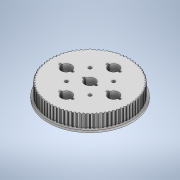
# Autodesk Inventor part: os_5_zebatka
Saved by Autodesk Inventor 2020.3 (Build 243373000, 373)
## iProperties
Created: 2021-03-12
Part Number: os_5_zebatka
Material: Generic
Document SubType Name: Modeling
Designer: patry
Density: 1 g/cm^3
Appearance: Default
Author: patry
Autodesk Inventor part; units mm, degrees
ref_plane "YZ Plane" through (0, 0, 0) normal (1, 0, 0) x (0, 1, 0)
ref_plane "XZ Plane" through (0, 0, 0) normal (0, 1, 0) x (-1, 0, 0)
ref_plane "XY Plane" through (0, 0, 0) normal (0, 0, 1) x (1, 0, 0)
sketch "Sketch1" plane through (0, 0, 0) normal (0, 1, 0) x (-1, 0, 0)
  circle A0 centre (0, 0) radius 40
  dimension "d0" = 80
  constraints: 1 centre point, 1 coincident
  measures "d0" diameter of A0
extrude "Extrusion1" add sketch "Sketch1" along normal blind 2
sketch "Sketch2" plane through (0, 2, 0) normal (0, 1, 0) x (1, 0, 0)
  circle A0 centre (0, 0) radius 38
  line L0 (0.3625, 37.9999) -> (-0.3625, 37.9999)
  arc A1 (-1.5, 36.8624) -> (-0.5625, 37.7999) centre (-1.5, 37.7999) ccw
  arc A2 (0.5625, 37.7999) -> (1.5, 36.8624) centre (1.5, 37.7999) ccw
  arc A3 (-0.3625, 37.9999) -> (-0.5625, 37.7999) centre (-0.3625, 37.7999) ccw
  arc A4 (0.5625, 37.7999) -> (0.3625, 37.9999) centre (0.3625, 37.7999) ccw
  arc A5 (-4.3876, 36.6311) -> (-3.5265, 37.6393) centre (-4.4611, 37.5657) ccw
  arc A6 (-3.3428, 37.8543) -> (-3.5265, 37.6393) centre (-3.3271, 37.655) ccw
  line L1 (-2.6201, 37.9112) -> (-3.3428, 37.8543)
  arc A7 (-2.405, 37.7275) -> (-2.6201, 37.9112) centre (-2.6044, 37.7118) ccw
  arc A8 (-2.405, 37.7275) -> (-1.3968, 36.8665) centre (-1.4704, 37.8011) ccw
  arc A9 (-7.2481, 36.1739) -> (-6.4688, 37.2465) centre (-7.3947, 37.0999) ccw
  arc A10 (-6.3025, 37.4754) -> (-6.4688, 37.2465) centre (-6.2712, 37.2778) ccw
  line L2 (-5.5865, 37.5888) -> (-6.3025, 37.4754)
  arc A11 (-5.3576, 37.4225) -> (-5.5865, 37.5888) centre (-5.5552, 37.3912) ccw
  arc A12 (-5.3576, 37.4225) -> (-4.285, 36.6432) centre (-4.4317, 37.5692) ccw
  arc A13 (-10.0639, 35.4937) -> (-9.3712, 36.6242) centre (-10.2828, 36.4053) ccw
  arc A14 (-9.2234, 36.8654) -> (-9.3712, 36.6242) centre (-9.1767, 36.6709) ccw
  line L3 (-8.5184, 37.0346) -> (-9.2234, 36.8654)
  arc A15 (-8.2773, 36.8868) -> (-8.5184, 37.0346) centre (-8.4717, 36.8401) ccw
  arc A16 (-8.2773, 36.8868) -> (-7.1468, 36.1941) centre (-7.3657, 37.1057) ccw
  arc A17 (-12.8177, 34.5947) -> (-12.2158, 35.776) centre (-13.1074, 35.4863) ccw
  arc A18 (-12.0874, 36.0281) -> (-12.2158, 35.776) centre (-12.0256, 35.8378) ccw
  line L4 (-11.3979, 36.2521) -> (-12.0874, 36.0281)
  arc A19 (-11.1458, 36.1237) -> (-11.3979, 36.2521) centre (-11.3361, 36.0619) ccw
  arc A20 (-11.1458, 36.1237) -> (-9.9645, 35.5218) centre (-10.2542, 36.4134) ccw
  arc A21 (-15.4925, 33.4824) -> (-14.9851, 34.7073) centre (-15.8512, 34.3485) ccw
  arc A22 (-14.8768, 34.9686) -> (-14.9851, 34.7073) centre (-14.8003, 34.7839) ccw
  line L5 (-14.207, 35.2461) -> (-14.8768, 34.9686)
  arc A23 (-13.9457, 35.1378) -> (-14.207, 35.2461) centre (-14.1305, 35.0613) ccw
  arc A24 (-13.9457, 35.1378) -> (-12.7208, 34.6305) centre (-13.0796, 35.4966) ccw
  arc A25 (-18.0717, 32.1637) -> (-17.662, 33.4246) centre (-18.4973, 32.999) ccw
  arc A26 (-17.5746, 33.6936) -> (-17.662, 33.4246) centre (-17.4838, 33.5154) ccw
  line L6 (-16.9286, 34.0227) -> (-17.5746, 33.6936)
  arc A27 (-16.6596, 33.9353) -> (-16.9286, 34.0227) centre (-16.8378, 33.8445) ccw
  arc A28 (-16.6596, 33.9353) -> (-15.3987, 33.5256) centre (-15.8243, 34.361) ccw
  arc A29 (-20.5395, 30.6466) -> (-20.23, 31.9358) centre (-21.0294, 31.446) ccw
  arc A30 (-20.164, 32.2109) -> (-20.23, 31.9358) centre (-20.0595, 32.0403) ccw
  line L7 (-19.5458, 32.5897) -> (-20.164, 32.2109)
  arc A31 (-19.2708, 32.5236) -> (-19.5458, 32.5897) centre (-19.4413, 32.4191) ccw
  arc A32 (-19.2708, 32.5236) -> (-17.9816, 32.2141) centre (-18.4714, 33.0135) ccw
  arc A33 (-22.8807, 28.9406) -> (-22.6733, 30.2501) centre (-23.4318, 29.6991) ccw
  arc A34 (-22.6291, 30.5295) -> (-22.6733, 30.2501) centre (-22.5115, 30.3677) ccw
  line L8 (-22.0425, 30.9557) -> (-22.6291, 30.5295)
  arc A35 (-21.7632, 30.9114) -> (-22.0425, 30.9557) centre (-21.925, 30.7939) ccw
  arc A36 (-21.7632, 30.9114) -> (-20.4537, 30.704) centre (-21.0047, 31.4625) ccw
  arc A37 (-25.0808, 27.0562) -> (-24.9768, 28.378) centre (-25.6897, 27.7691) ccw
  arc A38 (-24.9546, 28.6599) -> (-24.9768, 28.378) centre (-24.8247, 28.5079) ccw
  line L9 (-24.4033, 29.1308) -> (-24.9546, 28.6599)
  arc A39 (-24.1214, 29.1086) -> (-24.4033, 29.1308) centre (-24.2734, 28.9787) ccw
  arc A40 (-24.1214, 29.1086) -> (-22.7996, 29.0046) centre (-23.4085, 29.7175) ccw
  arc A41 (-27.1263, 25.005) -> (-27.1263, 26.3308) centre (-27.7892, 25.6679) ccw
  arc A42 (-27.1263, 26.6137) -> (-27.1263, 26.3308) centre (-26.9849, 26.4723) ccw
  line L10 (-26.6137, 27.1263) -> (-27.1263, 26.6137)
  arc A43 (-26.3308, 27.1263) -> (-26.6137, 27.1263) centre (-26.4723, 26.9849) ccw
  arc A44 (-26.3308, 27.1263) -> (-25.005, 27.1263) centre (-25.6679, 27.7892) ccw
  arc A45 (-29.0046, 22.7996) -> (-29.1086, 24.1214) centre (-29.7175, 23.4085) ccw
  arc A46 (-29.1308, 24.4033) -> (-29.1086, 24.1214) centre (-28.9787, 24.2734) ccw
  line L11 (-28.6599, 24.9546) -> (-29.1308, 24.4033)
  arc A47 (-28.378, 24.9768) -> (-28.6599, 24.9546) centre (-28.5079, 24.8247) ccw
  arc A48 (-28.378, 24.9768) -> (-27.0562, 25.0808) centre (-27.7691, 25.6897) ccw
  arc A49 (-30.704, 20.4537) -> (-30.9114, 21.7632) centre (-31.4625, 21.0047) ccw
  arc A50 (-30.9557, 22.0425) -> (-30.9114, 21.7632) centre (-30.7939, 21.925) ccw
  line L12 (-30.5295, 22.6291) -> (-30.9557, 22.0425)
  arc A51 (-30.2501, 22.6733) -> (-30.5295, 22.6291) centre (-30.3677, 22.5115) ccw
  arc A52 (-30.2501, 22.6733) -> (-28.9406, 22.8807) centre (-29.6991, 23.4318) ccw
  arc A53 (-32.2141, 17.9816) -> (-32.5236, 19.2708) centre (-33.0135, 18.4714) ccw
  arc A54 (-32.5897, 19.5458) -> (-32.5236, 19.2708) centre (-32.4191, 19.4413) ccw
  line L13 (-32.2109, 20.164) -> (-32.5897, 19.5458)
  arc A55 (-31.9358, 20.23) -> (-32.2109, 20.164) centre (-32.0403, 20.0595) ccw
  arc A56 (-31.9358, 20.23) -> (-30.6466, 20.5395) centre (-31.446, 21.0294) ccw
  arc A57 (-33.5256, 15.3987) -> (-33.9353, 16.6596) centre (-34.361, 15.8243) ccw
  arc A58 (-34.0227, 16.9286) -> (-33.9353, 16.6596) centre (-33.8445, 16.8378) ccw
  line L14 (-33.6936, 17.5746) -> (-34.0227, 16.9286)
  arc A59 (-33.4246, 17.662) -> (-33.6936, 17.5746) centre (-33.5154, 17.4838) ccw
  arc A60 (-33.4246, 17.662) -> (-32.1637, 18.0717) centre (-32.999, 18.4973) ccw
  arc A61 (-34.6305, 12.7208) -> (-35.1378, 13.9457) centre (-35.4966, 13.0796) ccw
  arc A62 (-35.2461, 14.207) -> (-35.1378, 13.9457) centre (-35.0613, 14.1305) ccw
  line L15 (-34.9686, 14.8768) -> (-35.2461, 14.207)
  arc A63 (-34.7073, 14.9851) -> (-34.9686, 14.8768) centre (-34.7839, 14.8003) ccw
  arc A64 (-34.7073, 14.9851) -> (-33.4824, 15.4925) centre (-34.3485, 15.8512) ccw
  arc A65 (-35.5218, 9.9645) -> (-36.1237, 11.1458) centre (-36.4134, 10.2542) ccw
  arc A66 (-36.2521, 11.3979) -> (-36.1237, 11.1458) centre (-36.0619, 11.3361) ccw
  line L16 (-36.0281, 12.0874) -> (-36.2521, 11.3979)
  arc A67 (-35.776, 12.2158) -> (-36.0281, 12.0874) centre (-35.8378, 12.0256) ccw
  arc A68 (-35.776, 12.2158) -> (-34.5947, 12.8177) centre (-35.4863, 13.1074) ccw
  arc A69 (-36.1941, 7.1468) -> (-36.8868, 8.2773) centre (-37.1057, 7.3657) ccw
  arc A70 (-37.0346, 8.5184) -> (-36.8868, 8.2773) centre (-36.8401, 8.4717) ccw
  line L17 (-36.8654, 9.2234) -> (-37.0346, 8.5184)
  arc A71 (-36.6242, 9.3712) -> (-36.8654, 9.2234) centre (-36.6709, 9.1767) ccw
  arc A72 (-36.6242, 9.3712) -> (-35.4937, 10.0639) centre (-36.4053, 10.2828) ccw
  arc A73 (-36.6432, 4.285) -> (-37.4225, 5.3576) centre (-37.5692, 4.4317) ccw
  arc A74 (-37.5888, 5.5865) -> (-37.4225, 5.3576) centre (-37.3912, 5.5552) ccw
  line L18 (-37.4754, 6.3025) -> (-37.5888, 5.5865)
  arc A75 (-37.2465, 6.4688) -> (-37.4754, 6.3025) centre (-37.2778, 6.2712) ccw
  arc A76 (-37.2465, 6.4688) -> (-36.1739, 7.2481) centre (-37.0999, 7.3947) ccw
  arc A77 (-36.8665, 1.3968) -> (-37.7275, 2.405) centre (-37.8011, 1.4704) ccw
  arc A78 (-37.9112, 2.6201) -> (-37.7275, 2.405) centre (-37.7118, 2.6044) ccw
  line L19 (-37.8543, 3.3428) -> (-37.9112, 2.6201)
  arc A79 (-37.6393, 3.5265) -> (-37.8543, 3.3428) centre (-37.655, 3.3271) ccw
  arc A80 (-37.6393, 3.5265) -> (-36.6311, 4.3876) centre (-37.5657, 4.4611) ccw
  arc A81 (-36.8624, -1.5) -> (-37.7999, -0.5625) centre (-37.7999, -1.5) ccw
  arc A82 (-37.9999, -0.3625) -> (-37.7999, -0.5625) centre (-37.7999, -0.3625) ccw
  line L20 (-37.9999, 0.3625) -> (-37.9999, -0.3625)
  arc A83 (-37.7999, 0.5625) -> (-37.9999, 0.3625) centre (-37.7999, 0.3625) ccw
  arc A84 (-37.7999, 0.5625) -> (-36.8624, 1.5) centre (-37.7999, 1.5) ccw
  arc A85 (-36.6311, -4.3876) -> (-37.6393, -3.5265) centre (-37.5657, -4.4611) ccw
  arc A86 (-37.8543, -3.3428) -> (-37.6393, -3.5265) centre (-37.655, -3.3271) ccw
  line L21 (-37.9112, -2.6201) -> (-37.8543, -3.3428)
  arc A87 (-37.7275, -2.405) -> (-37.9112, -2.6201) centre (-37.7118, -2.6044) ccw
  arc A88 (-37.7275, -2.405) -> (-36.8665, -1.3968) centre (-37.8011, -1.4704) ccw
  arc A89 (-36.1739, -7.2481) -> (-37.2465, -6.4688) centre (-37.0999, -7.3947) ccw
  arc A90 (-37.4754, -6.3025) -> (-37.2465, -6.4688) centre (-37.2778, -6.2712) ccw
  line L22 (-37.5888, -5.5865) -> (-37.4754, -6.3025)
  arc A91 (-37.4225, -5.3576) -> (-37.5888, -5.5865) centre (-37.3912, -5.5552) ccw
  arc A92 (-37.4225, -5.3576) -> (-36.6432, -4.285) centre (-37.5692, -4.4317) ccw
  arc A93 (-35.4937, -10.0639) -> (-36.6242, -9.3712) centre (-36.4053, -10.2828) ccw
  arc A94 (-36.8654, -9.2234) -> (-36.6242, -9.3712) centre (-36.6709, -9.1767) ccw
  line L23 (-37.0346, -8.5184) -> (-36.8654, -9.2234)
  arc A95 (-36.8868, -8.2773) -> (-37.0346, -8.5184) centre (-36.8401, -8.4717) ccw
  arc A96 (-36.8868, -8.2773) -> (-36.1941, -7.1468) centre (-37.1057, -7.3657) ccw
  arc A97 (-34.5947, -12.8177) -> (-35.776, -12.2158) centre (-35.4863, -13.1074) ccw
  arc A98 (-36.0281, -12.0874) -> (-35.776, -12.2158) centre (-35.8378, -12.0256) ccw
  line L24 (-36.2521, -11.3979) -> (-36.0281, -12.0874)
  arc A99 (-36.1237, -11.1458) -> (-36.2521, -11.3979) centre (-36.0619, -11.3361) ccw
  arc A100 (-36.1237, -11.1458) -> (-35.5218, -9.9645) centre (-36.4134, -10.2542) ccw
  arc A101 (-33.4824, -15.4925) -> (-34.7073, -14.9851) centre (-34.3485, -15.8512) ccw
  arc A102 (-34.9686, -14.8768) -> (-34.7073, -14.9851) centre (-34.7839, -14.8003) ccw
  line L25 (-35.2461, -14.207) -> (-34.9686, -14.8768)
  arc A103 (-35.1378, -13.9457) -> (-35.2461, -14.207) centre (-35.0613, -14.1305) ccw
  arc A104 (-35.1378, -13.9457) -> (-34.6305, -12.7208) centre (-35.4966, -13.0796) ccw
  arc A105 (-32.1637, -18.0717) -> (-33.4246, -17.662) centre (-32.999, -18.4973) ccw
  arc A106 (-33.6936, -17.5746) -> (-33.4246, -17.662) centre (-33.5154, -17.4838) ccw
  line L26 (-34.0227, -16.9286) -> (-33.6936, -17.5746)
  arc A107 (-33.9353, -16.6596) -> (-34.0227, -16.9286) centre (-33.8445, -16.8378) ccw
  arc A108 (-33.9353, -16.6596) -> (-33.5256, -15.3987) centre (-34.361, -15.8243) ccw
  arc A109 (-30.6466, -20.5395) -> (-31.9358, -20.23) centre (-31.446, -21.0294) ccw
  arc A110 (-32.2109, -20.164) -> (-31.9358, -20.23) centre (-32.0403, -20.0595) ccw
  line L27 (-32.5897, -19.5458) -> (-32.2109, -20.164)
  arc A111 (-32.5236, -19.2708) -> (-32.5897, -19.5458) centre (-32.4191, -19.4413) ccw
  arc A112 (-32.5236, -19.2708) -> (-32.2141, -17.9816) centre (-33.0135, -18.4714) ccw
  arc A113 (-28.9406, -22.8807) -> (-30.2501, -22.6733) centre (-29.6991, -23.4318) ccw
  arc A114 (-30.5295, -22.6291) -> (-30.2501, -22.6733) centre (-30.3677, -22.5115) ccw
  line L28 (-30.9557, -22.0425) -> (-30.5295, -22.6291)
  arc A115 (-30.9114, -21.7632) -> (-30.9557, -22.0425) centre (-30.7939, -21.925) ccw
  arc A116 (-30.9114, -21.7632) -> (-30.704, -20.4537) centre (-31.4625, -21.0047) ccw
  arc A117 (-27.0562, -25.0808) -> (-28.378, -24.9768) centre (-27.7691, -25.6897) ccw
  arc A118 (-28.6599, -24.9546) -> (-28.378, -24.9768) centre (-28.5079, -24.8247) ccw
  line L29 (-29.1308, -24.4033) -> (-28.6599, -24.9546)
  arc A119 (-29.1086, -24.1214) -> (-29.1308, -24.4033) centre (-28.9787, -24.2734) ccw
  arc A120 (-29.1086, -24.1214) -> (-29.0046, -22.7996) centre (-29.7175, -23.4085) ccw
  arc A121 (-25.005, -27.1263) -> (-26.3308, -27.1263) centre (-25.6679, -27.7892) ccw
  arc A122 (-26.6137, -27.1263) -> (-26.3308, -27.1263) centre (-26.4723, -26.9849) ccw
  line L30 (-27.1263, -26.6137) -> (-26.6137, -27.1263)
  arc A123 (-27.1263, -26.3308) -> (-27.1263, -26.6137) centre (-26.9849, -26.4723) ccw
  arc A124 (-27.1263, -26.3308) -> (-27.1263, -25.005) centre (-27.7892, -25.6679) ccw
  arc A125 (-22.7996, -29.0046) -> (-24.1214, -29.1086) centre (-23.4085, -29.7175) ccw
  arc A126 (-24.4033, -29.1308) -> (-24.1214, -29.1086) centre (-24.2734, -28.9787) ccw
  line L31 (-24.9546, -28.6599) -> (-24.4033, -29.1308)
  arc A127 (-24.9768, -28.378) -> (-24.9546, -28.6599) centre (-24.8247, -28.5079) ccw
  arc A128 (-24.9768, -28.378) -> (-25.0808, -27.0562) centre (-25.6897, -27.7691) ccw
  arc A129 (-20.4537, -30.704) -> (-21.7632, -30.9114) centre (-21.0047, -31.4625) ccw
  arc A130 (-22.0425, -30.9557) -> (-21.7632, -30.9114) centre (-21.925, -30.7939) ccw
  line L32 (-22.6291, -30.5295) -> (-22.0425, -30.9557)
  arc A131 (-22.6733, -30.2501) -> (-22.6291, -30.5295) centre (-22.5115, -30.3677) ccw
  arc A132 (-22.6733, -30.2501) -> (-22.8807, -28.9406) centre (-23.4318, -29.6991) ccw
  arc A133 (-17.9816, -32.2141) -> (-19.2708, -32.5236) centre (-18.4714, -33.0135) ccw
  arc A134 (-19.5458, -32.5897) -> (-19.2708, -32.5236) centre (-19.4413, -32.4191) ccw
  line L33 (-20.164, -32.2109) -> (-19.5458, -32.5897)
  arc A135 (-20.23, -31.9358) -> (-20.164, -32.2109) centre (-20.0595, -32.0403) ccw
  arc A136 (-20.23, -31.9358) -> (-20.5395, -30.6466) centre (-21.0294, -31.446) ccw
  arc A137 (-15.3987, -33.5256) -> (-16.6596, -33.9353) centre (-15.8243, -34.361) ccw
  arc A138 (-16.9286, -34.0227) -> (-16.6596, -33.9353) centre (-16.8378, -33.8445) ccw
  line L34 (-17.5746, -33.6936) -> (-16.9286, -34.0227)
  arc A139 (-17.662, -33.4246) -> (-17.5746, -33.6936) centre (-17.4838, -33.5154) ccw
  arc A140 (-17.662, -33.4246) -> (-18.0717, -32.1637) centre (-18.4973, -32.999) ccw
  arc A141 (-12.7208, -34.6305) -> (-13.9457, -35.1378) centre (-13.0796, -35.4966) ccw
  arc A142 (-14.207, -35.2461) -> (-13.9457, -35.1378) centre (-14.1305, -35.0613) ccw
  line L35 (-14.8768, -34.9686) -> (-14.207, -35.2461)
  arc A143 (-14.9851, -34.7073) -> (-14.8768, -34.9686) centre (-14.8003, -34.7839) ccw
  arc A144 (-14.9851, -34.7073) -> (-15.4925, -33.4824) centre (-15.8512, -34.3485) ccw
  arc A145 (-9.9645, -35.5218) -> (-11.1458, -36.1237) centre (-10.2542, -36.4134) ccw
  arc A146 (-11.3979, -36.2521) -> (-11.1458, -36.1237) centre (-11.3361, -36.0619) ccw
  line L36 (-12.0874, -36.0281) -> (-11.3979, -36.2521)
  arc A147 (-12.2158, -35.776) -> (-12.0874, -36.0281) centre (-12.0256, -35.8378) ccw
  arc A148 (-12.2158, -35.776) -> (-12.8177, -34.5947) centre (-13.1074, -35.4863) ccw
  arc A149 (-7.1468, -36.1941) -> (-8.2773, -36.8868) centre (-7.3657, -37.1057) ccw
  arc A150 (-8.5184, -37.0346) -> (-8.2773, -36.8868) centre (-8.4717, -36.8401) ccw
  line L37 (-9.2234, -36.8654) -> (-8.5184, -37.0346)
  arc A151 (-9.3712, -36.6242) -> (-9.2234, -36.8654) centre (-9.1767, -36.6709) ccw
  arc A152 (-9.3712, -36.6242) -> (-10.0639, -35.4937) centre (-10.2828, -36.4053) ccw
  arc A153 (-4.285, -36.6432) -> (-5.3576, -37.4225) centre (-4.4317, -37.5692) ccw
  arc A154 (-5.5865, -37.5888) -> (-5.3576, -37.4225) centre (-5.5552, -37.3912) ccw
  line L38 (-6.3025, -37.4754) -> (-5.5865, -37.5888)
  arc A155 (-6.4688, -37.2465) -> (-6.3025, -37.4754) centre (-6.2712, -37.2778) ccw
  arc A156 (-6.4688, -37.2465) -> (-7.2481, -36.1739) centre (-7.3947, -37.0999) ccw
  arc A157 (-1.3968, -36.8665) -> (-2.405, -37.7275) centre (-1.4704, -37.8011) ccw
  arc A158 (-2.6201, -37.9112) -> (-2.405, -37.7275) centre (-2.6044, -37.7118) ccw
  line L39 (-3.3428, -37.8543) -> (-2.6201, -37.9112)
  arc A159 (-3.5265, -37.6393) -> (-3.3428, -37.8543) centre (-3.3271, -37.655) ccw
  arc A160 (-3.5265, -37.6393) -> (-4.3876, -36.6311) centre (-4.4611, -37.5657) ccw
  arc A161 (1.5, -36.8624) -> (0.5625, -37.7999) centre (1.5, -37.7999) ccw
  arc A162 (0.3625, -37.9999) -> (0.5625, -37.7999) centre (0.3625, -37.7999) ccw
  line L40 (-0.3625, -37.9999) -> (0.3625, -37.9999)
  arc A163 (-0.5625, -37.7999) -> (-0.3625, -37.9999) centre (-0.3625, -37.7999) ccw
  arc A164 (-0.5625, -37.7999) -> (-1.5, -36.8624) centre (-1.5, -37.7999) ccw
  arc A165 (4.3876, -36.6311) -> (3.5265, -37.6393) centre (4.4611, -37.5657) ccw
  arc A166 (3.3428, -37.8543) -> (3.5265, -37.6393) centre (3.3271, -37.655) ccw
  line L41 (2.6201, -37.9112) -> (3.3428, -37.8543)
  arc A167 (2.405, -37.7275) -> (2.6201, -37.9112) centre (2.6044, -37.7118) ccw
  arc A168 (2.405, -37.7275) -> (1.3968, -36.8665) centre (1.4704, -37.8011) ccw
  arc A169 (7.2481, -36.1739) -> (6.4688, -37.2465) centre (7.3947, -37.0999) ccw
  arc A170 (6.3025, -37.4754) -> (6.4688, -37.2465) centre (6.2712, -37.2778) ccw
  line L42 (5.5865, -37.5888) -> (6.3025, -37.4754)
  arc A171 (5.3576, -37.4225) -> (5.5865, -37.5888) centre (5.5552, -37.3912) ccw
  arc A172 (5.3576, -37.4225) -> (4.285, -36.6432) centre (4.4317, -37.5692) ccw
  arc A173 (10.0639, -35.4937) -> (9.3712, -36.6242) centre (10.2828, -36.4053) ccw
  arc A174 (9.2234, -36.8654) -> (9.3712, -36.6242) centre (9.1767, -36.6709) ccw
  line L43 (8.5184, -37.0346) -> (9.2234, -36.8654)
  arc A175 (8.2773, -36.8868) -> (8.5184, -37.0346) centre (8.4717, -36.8401) ccw
  arc A176 (8.2773, -36.8868) -> (7.1468, -36.1941) centre (7.3657, -37.1057) ccw
  arc A177 (12.8177, -34.5947) -> (12.2158, -35.776) centre (13.1074, -35.4863) ccw
  arc A178 (12.0874, -36.0281) -> (12.2158, -35.776) centre (12.0256, -35.8378) ccw
  line L44 (11.3979, -36.2521) -> (12.0874, -36.0281)
  arc A179 (11.1458, -36.1237) -> (11.3979, -36.2521) centre (11.3361, -36.0619) ccw
  arc A180 (11.1458, -36.1237) -> (9.9645, -35.5218) centre (10.2542, -36.4134) ccw
  arc A181 (15.4925, -33.4824) -> (14.9851, -34.7073) centre (15.8512, -34.3485) ccw
  arc A182 (14.8768, -34.9686) -> (14.9851, -34.7073) centre (14.8003, -34.7839) ccw
  line L45 (14.207, -35.2461) -> (14.8768, -34.9686)
  arc A183 (13.9457, -35.1378) -> (14.207, -35.2461) centre (14.1305, -35.0613) ccw
  arc A184 (13.9457, -35.1378) -> (12.7208, -34.6305) centre (13.0796, -35.4966) ccw
  arc A185 (18.0717, -32.1637) -> (17.662, -33.4246) centre (18.4973, -32.999) ccw
  arc A186 (17.5746, -33.6936) -> (17.662, -33.4246) centre (17.4838, -33.5154) ccw
  line L46 (16.9286, -34.0227) -> (17.5746, -33.6936)
  arc A187 (16.6596, -33.9353) -> (16.9286, -34.0227) centre (16.8378, -33.8445) ccw
  arc A188 (16.6596, -33.9353) -> (15.3987, -33.5256) centre (15.8243, -34.361) ccw
  arc A189 (20.5395, -30.6466) -> (20.23, -31.9358) centre (21.0294, -31.446) ccw
  arc A190 (20.164, -32.2109) -> (20.23, -31.9358) centre (20.0595, -32.0403) ccw
  line L47 (19.5458, -32.5897) -> (20.164, -32.2109)
  arc A191 (19.2708, -32.5236) -> (19.5458, -32.5897) centre (19.4413, -32.4191) ccw
  arc A192 (19.2708, -32.5236) -> (17.9816, -32.2141) centre (18.4714, -33.0135) ccw
  arc A193 (22.8807, -28.9406) -> (22.6733, -30.2501) centre (23.4318, -29.6991) ccw
  arc A194 (22.6291, -30.5295) -> (22.6733, -30.2501) centre (22.5115, -30.3677) ccw
  line L48 (22.0425, -30.9557) -> (22.6291, -30.5295)
  arc A195 (21.7632, -30.9114) -> (22.0425, -30.9557) centre (21.925, -30.7939) ccw
  arc A196 (21.7632, -30.9114) -> (20.4537, -30.704) centre (21.0047, -31.4625) ccw
  arc A197 (25.0808, -27.0562) -> (24.9768, -28.378) centre (25.6897, -27.7691) ccw
  arc A198 (24.9546, -28.6599) -> (24.9768, -28.378) centre (24.8247, -28.5079) ccw
  line L49 (24.4033, -29.1308) -> (24.9546, -28.6599)
  arc A199 (24.1214, -29.1086) -> (24.4033, -29.1308) centre (24.2734, -28.9787) ccw
  arc A200 (24.1214, -29.1086) -> (22.7996, -29.0046) centre (23.4085, -29.7175) ccw
  arc A201 (27.1263, -25.005) -> (27.1263, -26.3308) centre (27.7892, -25.6679) ccw
  arc A202 (27.1263, -26.6137) -> (27.1263, -26.3308) centre (26.9849, -26.4723) ccw
  line L50 (26.6137, -27.1263) -> (27.1263, -26.6137)
  arc A203 (26.3308, -27.1263) -> (26.6137, -27.1263) centre (26.4723, -26.9849) ccw
  arc A204 (26.3308, -27.1263) -> (25.005, -27.1263) centre (25.6679, -27.7892) ccw
  arc A205 (29.0046, -22.7996) -> (29.1086, -24.1214) centre (29.7175, -23.4085) ccw
  arc A206 (29.1308, -24.4033) -> (29.1086, -24.1214) centre (28.9787, -24.2734) ccw
  line L51 (28.6599, -24.9546) -> (29.1308, -24.4033)
  arc A207 (28.378, -24.9768) -> (28.6599, -24.9546) centre (28.5079, -24.8247) ccw
  arc A208 (28.378, -24.9768) -> (27.0562, -25.0808) centre (27.7691, -25.6897) ccw
  arc A209 (30.704, -20.4537) -> (30.9114, -21.7632) centre (31.4625, -21.0047) ccw
  arc A210 (30.9557, -22.0425) -> (30.9114, -21.7632) centre (30.7939, -21.925) ccw
  line L52 (30.5295, -22.6291) -> (30.9557, -22.0425)
  arc A211 (30.2501, -22.6733) -> (30.5295, -22.6291) centre (30.3677, -22.5115) ccw
  arc A212 (30.2501, -22.6733) -> (28.9406, -22.8807) centre (29.6991, -23.4318) ccw
  arc A213 (32.2141, -17.9816) -> (32.5236, -19.2708) centre (33.0135, -18.4714) ccw
  arc A214 (32.5897, -19.5458) -> (32.5236, -19.2708) centre (32.4191, -19.4413) ccw
  line L53 (32.2109, -20.164) -> (32.5897, -19.5458)
  arc A215 (31.9358, -20.23) -> (32.2109, -20.164) centre (32.0403, -20.0595) ccw
  arc A216 (31.9358, -20.23) -> (30.6466, -20.5395) centre (31.446, -21.0294) ccw
  arc A217 (33.5256, -15.3987) -> (33.9353, -16.6596) centre (34.361, -15.8243) ccw
  arc A218 (34.0227, -16.9286) -> (33.9353, -16.6596) centre (33.8445, -16.8378) ccw
  line L54 (33.6936, -17.5746) -> (34.0227, -16.9286)
  arc A219 (33.4246, -17.662) -> (33.6936, -17.5746) centre (33.5154, -17.4838) ccw
  arc A220 (33.4246, -17.662) -> (32.1637, -18.0717) centre (32.999, -18.4973) ccw
  arc A221 (34.6305, -12.7208) -> (35.1378, -13.9457) centre (35.4966, -13.0796) ccw
  arc A222 (35.2461, -14.207) -> (35.1378, -13.9457) centre (35.0613, -14.1305) ccw
  line L55 (34.9686, -14.8768) -> (35.2461, -14.207)
  arc A223 (34.7073, -14.9851) -> (34.9686, -14.8768) centre (34.7839, -14.8003) ccw
  arc A224 (34.7073, -14.9851) -> (33.4824, -15.4925) centre (34.3485, -15.8512) ccw
  arc A225 (35.5218, -9.9645) -> (36.1237, -11.1458) centre (36.4134, -10.2542) ccw
  arc A226 (36.2521, -11.3979) -> (36.1237, -11.1458) centre (36.0619, -11.3361) ccw
  line L56 (36.0281, -12.0874) -> (36.2521, -11.3979)
  arc A227 (35.776, -12.2158) -> (36.0281, -12.0874) centre (35.8378, -12.0256) ccw
  arc A228 (35.776, -12.2158) -> (34.5947, -12.8177) centre (35.4863, -13.1074) ccw
  arc A229 (36.1941, -7.1468) -> (36.8868, -8.2773) centre (37.1057, -7.3657) ccw
  arc A230 (37.0346, -8.5184) -> (36.8868, -8.2773) centre (36.8401, -8.4717) ccw
  line L57 (36.8654, -9.2234) -> (37.0346, -8.5184)
  arc A231 (36.6242, -9.3712) -> (36.8654, -9.2234) centre (36.6709, -9.1767) ccw
  arc A232 (36.6242, -9.3712) -> (35.4937, -10.0639) centre (36.4053, -10.2828) ccw
  arc A233 (36.6432, -4.285) -> (37.4225, -5.3576) centre (37.5692, -4.4317) ccw
  arc A234 (37.5888, -5.5865) -> (37.4225, -5.3576) centre (37.3912, -5.5552) ccw
  line L58 (37.4754, -6.3025) -> (37.5888, -5.5865)
  arc A235 (37.2465, -6.4688) -> (37.4754, -6.3025) centre (37.2778, -6.2712) ccw
  arc A236 (37.2465, -6.4688) -> (36.1739, -7.2481) centre (37.0999, -7.3947) ccw
  arc A237 (36.8665, -1.3968) -> (37.7275, -2.405) centre (37.8011, -1.4704) ccw
  arc A238 (37.9112, -2.6201) -> (37.7275, -2.405) centre (37.7118, -2.6044) ccw
  line L59 (37.8543, -3.3428) -> (37.9112, -2.6201)
  arc A239 (37.6393, -3.5265) -> (37.8543, -3.3428) centre (37.655, -3.3271) ccw
  arc A240 (37.6393, -3.5265) -> (36.6311, -4.3876) centre (37.5657, -4.4611) ccw
  arc A241 (36.8624, 1.5) -> (37.7999, 0.5625) centre (37.7999, 1.5) ccw
  arc A242 (37.9999, 0.3625) -> (37.7999, 0.5625) centre (37.7999, 0.3625) ccw
  line L60 (37.9999, -0.3625) -> (37.9999, 0.3625)
  arc A243 (37.7999, -0.5625) -> (37.9999, -0.3625) centre (37.7999, -0.3625) ccw
  arc A244 (37.7999, -0.5625) -> (36.8624, -1.5) centre (37.7999, -1.5) ccw
  arc A245 (36.6311, 4.3876) -> (37.6393, 3.5265) centre (37.5657, 4.4611) ccw
  arc A246 (37.8543, 3.3428) -> (37.6393, 3.5265) centre (37.655, 3.3271) ccw
  line L61 (37.9112, 2.6201) -> (37.8543, 3.3428)
  arc A247 (37.7275, 2.405) -> (37.9112, 2.6201) centre (37.7118, 2.6044) ccw
  arc A248 (37.7275, 2.405) -> (36.8665, 1.3968) centre (37.8011, 1.4704) ccw
  arc A249 (36.1739, 7.2481) -> (37.2465, 6.4688) centre (37.0999, 7.3947) ccw
  arc A250 (37.4754, 6.3025) -> (37.2465, 6.4688) centre (37.2778, 6.2712) ccw
  line L62 (37.5888, 5.5865) -> (37.4754, 6.3025)
  arc A251 (37.4225, 5.3576) -> (37.5888, 5.5865) centre (37.3912, 5.5552) ccw
  arc A252 (37.4225, 5.3576) -> (36.6432, 4.285) centre (37.5692, 4.4317) ccw
  arc A253 (35.4937, 10.0639) -> (36.6242, 9.3712) centre (36.4053, 10.2828) ccw
  arc A254 (36.8654, 9.2234) -> (36.6242, 9.3712) centre (36.6709, 9.1767) ccw
  line L63 (37.0346, 8.5184) -> (36.8654, 9.2234)
  arc A255 (36.8868, 8.2773) -> (37.0346, 8.5184) centre (36.8401, 8.4717) ccw
  arc A256 (36.8868, 8.2773) -> (36.1941, 7.1468) centre (37.1057, 7.3657) ccw
  arc A257 (34.5947, 12.8177) -> (35.776, 12.2158) centre (35.4863, 13.1074) ccw
  arc A258 (36.0281, 12.0874) -> (35.776, 12.2158) centre (35.8378, 12.0256) ccw
  line L64 (36.2521, 11.3979) -> (36.0281, 12.0874)
  arc A259 (36.1237, 11.1458) -> (36.2521, 11.3979) centre (36.0619, 11.3361) ccw
  arc A260 (36.1237, 11.1458) -> (35.5218, 9.9645) centre (36.4134, 10.2542) ccw
  arc A261 (33.4824, 15.4925) -> (34.7073, 14.9851) centre (34.3485, 15.8512) ccw
  arc A262 (34.9686, 14.8768) -> (34.7073, 14.9851) centre (34.7839, 14.8003) ccw
  line L65 (35.2461, 14.207) -> (34.9686, 14.8768)
  arc A263 (35.1378, 13.9457) -> (35.2461, 14.207) centre (35.0613, 14.1305) ccw
  arc A264 (35.1378, 13.9457) -> (34.6305, 12.7208) centre (35.4966, 13.0796) ccw
  arc A265 (32.1637, 18.0717) -> (33.4246, 17.662) centre (32.999, 18.4973) ccw
  arc A266 (33.6936, 17.5746) -> (33.4246, 17.662) centre (33.5154, 17.4838) ccw
  line L66 (34.0227, 16.9286) -> (33.6936, 17.5746)
  arc A267 (33.9353, 16.6596) -> (34.0227, 16.9286) centre (33.8445, 16.8378) ccw
  arc A268 (33.9353, 16.6596) -> (33.5256, 15.3987) centre (34.361, 15.8243) ccw
  arc A269 (30.6466, 20.5395) -> (31.9358, 20.23) centre (31.446, 21.0294) ccw
  arc A270 (32.2109, 20.164) -> (31.9358, 20.23) centre (32.0403, 20.0595) ccw
  line L67 (32.5897, 19.5458) -> (32.2109, 20.164)
  arc A271 (32.5236, 19.2708) -> (32.5897, 19.5458) centre (32.4191, 19.4413) ccw
  arc A272 (32.5236, 19.2708) -> (32.2141, 17.9816) centre (33.0135, 18.4714) ccw
  arc A273 (28.9406, 22.8807) -> (30.2501, 22.6733) centre (29.6991, 23.4318) ccw
  arc A274 (30.5295, 22.6291) -> (30.2501, 22.6733) centre (30.3677, 22.5115) ccw
  line L68 (30.9557, 22.0425) -> (30.5295, 22.6291)
  arc A275 (30.9114, 21.7632) -> (30.9557, 22.0425) centre (30.7939, 21.925) ccw
  arc A276 (30.9114, 21.7632) -> (30.704, 20.4537) centre (31.4625, 21.0047) ccw
  arc A277 (27.0562, 25.0808) -> (28.378, 24.9768) centre (27.7691, 25.6897) ccw
  arc A278 (28.6599, 24.9546) -> (28.378, 24.9768) centre (28.5079, 24.8247) ccw
  line L69 (29.1308, 24.4033) -> (28.6599, 24.9546)
  arc A279 (29.1086, 24.1214) -> (29.1308, 24.4033) centre (28.9787, 24.2734) ccw
  arc A280 (29.1086, 24.1214) -> (29.0046, 22.7996) centre (29.7175, 23.4085) ccw
  arc A281 (25.005, 27.1263) -> (26.3308, 27.1263) centre (25.6679, 27.7892) ccw
  arc A282 (26.6137, 27.1263) -> (26.3308, 27.1263) centre (26.4723, 26.9849) ccw
  line L70 (27.1263, 26.6137) -> (26.6137, 27.1263)
  arc A283 (27.1263, 26.3308) -> (27.1263, 26.6137) centre (26.9849, 26.4723) ccw
  arc A284 (27.1263, 26.3308) -> (27.1263, 25.005) centre (27.7892, 25.6679) ccw
  arc A285 (22.7996, 29.0046) -> (24.1214, 29.1086) centre (23.4085, 29.7175) ccw
  arc A286 (24.4033, 29.1308) -> (24.1214, 29.1086) centre (24.2734, 28.9787) ccw
  line L71 (24.9546, 28.6599) -> (24.4033, 29.1308)
  arc A287 (24.9768, 28.378) -> (24.9546, 28.6599) centre (24.8247, 28.5079) ccw
  arc A288 (24.9768, 28.378) -> (25.0808, 27.0562) centre (25.6897, 27.7691) ccw
  arc A289 (20.4537, 30.704) -> (21.7632, 30.9114) centre (21.0047, 31.4625) ccw
  arc A290 (22.0425, 30.9557) -> (21.7632, 30.9114) centre (21.925, 30.7939) ccw
  line L72 (22.6291, 30.5295) -> (22.0425, 30.9557)
  arc A291 (22.6733, 30.2501) -> (22.6291, 30.5295) centre (22.5115, 30.3677) ccw
  arc A292 (22.6733, 30.2501) -> (22.8807, 28.9406) centre (23.4318, 29.6991) ccw
  arc A293 (17.9816, 32.2141) -> (19.2708, 32.5236) centre (18.4714, 33.0135) ccw
  arc A294 (19.5458, 32.5897) -> (19.2708, 32.5236) centre (19.4413, 32.4191) ccw
  line L73 (20.164, 32.2109) -> (19.5458, 32.5897)
  arc A295 (20.23, 31.9358) -> (20.164, 32.2109) centre (20.0595, 32.0403) ccw
  arc A296 (20.23, 31.9358) -> (20.5395, 30.6466) centre (21.0294, 31.446) ccw
  arc A297 (15.3987, 33.5256) -> (16.6596, 33.9353) centre (15.8243, 34.361) ccw
  arc A298 (16.9286, 34.0227) -> (16.6596, 33.9353) centre (16.8378, 33.8445) ccw
  line L74 (17.5746, 33.6936) -> (16.9286, 34.0227)
  arc A299 (17.662, 33.4246) -> (17.5746, 33.6936) centre (17.4838, 33.5154) ccw
  arc A300 (17.662, 33.4246) -> (18.0717, 32.1637) centre (18.4973, 32.999) ccw
  arc A301 (12.7208, 34.6305) -> (13.9457, 35.1378) centre (13.0796, 35.4966) ccw
  arc A302 (14.207, 35.2461) -> (13.9457, 35.1378) centre (14.1305, 35.0613) ccw
  line L75 (14.8768, 34.9686) -> (14.207, 35.2461)
  arc A303 (14.9851, 34.7073) -> (14.8768, 34.9686) centre (14.8003, 34.7839) ccw
  arc A304 (14.9851, 34.7073) -> (15.4925, 33.4824) centre (15.8512, 34.3485) ccw
  arc A305 (9.9645, 35.5218) -> (11.1458, 36.1237) centre (10.2542, 36.4134) ccw
  arc A306 (11.3979, 36.2521) -> (11.1458, 36.1237) centre (11.3361, 36.0619) ccw
  line L76 (12.0874, 36.0281) -> (11.3979, 36.2521)
  arc A307 (12.2158, 35.776) -> (12.0874, 36.0281) centre (12.0256, 35.8378) ccw
  arc A308 (12.2158, 35.776) -> (12.8177, 34.5947) centre (13.1074, 35.4863) ccw
  arc A309 (7.1468, 36.1941) -> (8.2773, 36.8868) centre (7.3657, 37.1057) ccw
  arc A310 (8.5184, 37.0346) -> (8.2773, 36.8868) centre (8.4717, 36.8401) ccw
  line L77 (9.2234, 36.8654) -> (8.5184, 37.0346)
  arc A311 (9.3712, 36.6242) -> (9.2234, 36.8654) centre (9.1767, 36.6709) ccw
  arc A312 (9.3712, 36.6242) -> (10.0639, 35.4937) centre (10.2828, 36.4053) ccw
  arc A313 (4.285, 36.6432) -> (5.3576, 37.4225) centre (4.4317, 37.5692) ccw
  arc A314 (5.5865, 37.5888) -> (5.3576, 37.4225) centre (5.5552, 37.3912) ccw
  line L78 (6.3025, 37.4754) -> (5.5865, 37.5888)
  arc A315 (6.4688, 37.2465) -> (6.3025, 37.4754) centre (6.2712, 37.2778) ccw
  arc A316 (6.4688, 37.2465) -> (7.2481, 36.1739) centre (7.3947, 37.0999) ccw
  arc A317 (1.3968, 36.8665) -> (2.405, 37.7275) centre (1.4704, 37.8011) ccw
  arc A318 (2.6201, 37.9112) -> (2.405, 37.7275) centre (2.6044, 37.7118) ccw
  line L79 (3.3428, 37.8543) -> (2.6201, 37.9112)
  arc A319 (3.5265, 37.6393) -> (3.3428, 37.8543) centre (3.3271, 37.655) ccw
  arc A320 (3.5265, 37.6393) -> (4.3876, 36.6311) centre (4.4611, 37.5657) ccw
  point P0 (4.3362, 36.6366)
  point P1 (3.3703, 37.8502)
  point P2 (3.0584, 37.8767)
  point P3 (2.9045, 37.8888)
  point P4 (2.5923, 37.9115)
  point P5 (1.4484, 36.8638)
  point P6 (0.3902, 37.998)
  point P7 (0.0772, 37.9999)
  point P8 (-0.0772, 37.9999)
  point P9 (-0.3902, 37.998)
  point P10 (-1.4484, 36.8638)
  point P11 (-2.5923, 37.9115)
  point P12 (-2.9045, 37.8888)
  point P13 (-3.0584, 37.8767)
  point P14 (-3.3703, 37.8502)
  point P15 (-4.3362, 36.6366)
  point P16 (-5.5588, 37.5912)
  point P17 (-5.8682, 37.5442)
  point P18 (-6.0207, 37.52)
  point P19 (-6.3296, 37.4691)
  point P20 (-7.1973, 36.1834)
  point P21 (-8.4911, 37.0392)
  point P22 (-8.7958, 36.968)
  point P23 (-8.946, 36.932)
  point P24 (-9.2499, 36.857)
  point P25 (-10.0141, 35.5072)
  point P26 (-11.3709, 36.2588)
  point P27 (-11.6692, 36.1639)
  point P28 (-11.816, 36.1162)
  point P29 (-12.1131, 36.0177)
  point P30 (-12.769, 34.612)
  point P31 (-14.1807, 35.2549)
  point P32 (-14.4706, 35.1369)
  point P33 (-14.6133, 35.0778)
  point P34 (-14.9017, 34.9563)
  point P35 (-15.4453, 33.5035)
  point P36 (-16.9031, 34.0336)
  point P37 (-17.1828, 33.8932)
  point P38 (-17.3204, 33.8231)
  point P39 (-17.5984, 33.6793)
  point P40 (-18.0264, 32.1884)
  point P41 (-19.5212, 32.6025)
  point P42 (-19.7891, 32.4406)
  point P43 (-19.9207, 32.3599)
  point P44 (-20.1866, 32.1947)
  point P45 (-20.4963, 30.6748)
  point P46 (-22.019, 30.9704)
  point P47 (-22.2733, 30.788)
  point P48 (-22.3983, 30.6972)
  point P49 (-22.6503, 30.5117)
  point P50 (-22.8398, 28.9721)
  point P51 (-24.381, 29.1473)
  point P52 (-24.6203, 28.9455)
  point P53 (-24.7377, 28.8452)
  point P54 (-24.9744, 28.6405)
  point P55 (-25.0425, 27.0908)
  point P56 (-26.5927, 27.1445)
  point P57 (-26.8154, 26.9246)
  point P58 (-26.9246, 26.8154)
  point P59 (-27.1445, 26.5927)
  point P60 (-27.0908, 25.0425)
  point P61 (-28.6405, 24.9744)
  point P62 (-28.8452, 24.7377)
  point P63 (-28.9455, 24.6203)
  point P64 (-29.1473, 24.381)
  point P65 (-28.9721, 22.8398)
  point P66 (-30.5117, 22.6503)
  point P67 (-30.6972, 22.3983)
  point P68 (-30.788, 22.2733)
  point P69 (-30.9704, 22.019)
  point P70 (-30.6748, 20.4963)
  point P71 (-32.1947, 20.1866)
  point P72 (-32.3599, 19.9207)
  point P73 (-32.4406, 19.7891)
  point P74 (-32.6025, 19.5212)
  point P75 (-32.1884, 18.0264)
  point P76 (-33.6793, 17.5984)
  point P77 (-33.8231, 17.3204)
  point P78 (-33.8932, 17.1828)
  point P79 (-34.0336, 16.9031)
  point P80 (-33.5035, 15.4453)
  point P81 (-34.9563, 14.9017)
  point P82 (-35.0778, 14.6133)
  point P83 (-35.1369, 14.4706)
  point P84 (-35.2549, 14.1807)
  point P85 (-34.612, 12.769)
  point P86 (-36.0177, 12.1131)
  point P87 (-36.1162, 11.816)
  point P88 (-36.1639, 11.6692)
  point P89 (-36.2588, 11.3709)
  point P90 (-35.5072, 10.0141)
  point P91 (-36.857, 9.2499)
  point P92 (-36.932, 8.946)
  point P93 (-36.968, 8.7958)
  point P94 (-37.0392, 8.4911)
  point P95 (-36.1834, 7.1973)
  point P96 (-37.4691, 6.3296)
  point P97 (-37.52, 6.0207)
  point P98 (-37.5442, 5.8682)
  point P99 (-37.5912, 5.5588)
  point P100 (-36.6366, 4.3362)
  point P101 (-37.8502, 3.3703)
  point P102 (-37.8767, 3.0584)
  point P103 (-37.8888, 2.9045)
  point P104 (-37.9115, 2.5923)
  point P105 (-36.8638, 1.4484)
  point P106 (-37.998, 0.3902)
  point P107 (-37.9999, 0.0772)
  point P108 (-37.9999, -0.0772)
  point P109 (-37.998, -0.3902)
  point P110 (-36.8638, -1.4484)
  point P111 (-37.9115, -2.5923)
  point P112 (-37.8888, -2.9045)
  point P113 (-37.8767, -3.0584)
  point P114 (-37.8502, -3.3703)
  point P115 (-36.6366, -4.3362)
  point P116 (-37.5912, -5.5588)
  point P117 (-37.5442, -5.8682)
  point P118 (-37.52, -6.0207)
  point P119 (-37.4691, -6.3296)
  point P120 (-36.1834, -7.1973)
  point P121 (-37.0392, -8.4911)
  point P122 (-36.968, -8.7958)
  point P123 (-36.932, -8.946)
  point P124 (-36.857, -9.2499)
  point P125 (-35.5072, -10.0141)
  point P126 (-36.2588, -11.3709)
  point P127 (-36.1639, -11.6692)
  point P128 (-36.1162, -11.816)
  point P129 (-36.0177, -12.1131)
  point P130 (-34.612, -12.769)
  point P131 (-35.2549, -14.1807)
  point P132 (-35.1369, -14.4706)
  point P133 (-35.0778, -14.6133)
  point P134 (-34.9563, -14.9017)
  point P135 (-33.5035, -15.4453)
  point P136 (-34.0336, -16.9031)
  point P137 (-33.8932, -17.1828)
  point P138 (-33.8231, -17.3204)
  point P139 (-33.6793, -17.5984)
  point P140 (-32.1884, -18.0264)
  point P141 (-32.6025, -19.5212)
  point P142 (-32.4406, -19.7891)
  point P143 (-32.3599, -19.9207)
  point P144 (-32.1947, -20.1866)
  point P145 (-30.6748, -20.4963)
  point P146 (-30.9704, -22.019)
  point P147 (-30.788, -22.2733)
  point P148 (-30.6972, -22.3983)
  point P149 (-30.5117, -22.6503)
  point P150 (-28.9721, -22.8398)
  point P151 (-29.1473, -24.381)
  point P152 (-28.9455, -24.6203)
  point P153 (-28.8452, -24.7377)
  point P154 (-28.6405, -24.9744)
  point P155 (-27.0908, -25.0425)
  point P156 (-27.1445, -26.5927)
  point P157 (-26.9246, -26.8154)
  point P158 (-26.8154, -26.9246)
  point P159 (-26.5927, -27.1445)
  point P160 (-25.0425, -27.0908)
  point P161 (-24.9744, -28.6405)
  point P162 (-24.7377, -28.8452)
  point P163 (-24.6203, -28.9455)
  point P164 (-24.381, -29.1473)
  point P165 (-22.8398, -28.9721)
  point P166 (-22.6503, -30.5117)
  point P167 (-22.3983, -30.6972)
  point P168 (-22.2733, -30.788)
  point P169 (-22.019, -30.9704)
  point P170 (-20.4963, -30.6748)
  point P171 (-20.1866, -32.1947)
  point P172 (-19.9207, -32.3599)
  point P173 (-19.7891, -32.4406)
  point P174 (-19.5212, -32.6025)
  point P175 (-18.0264, -32.1884)
  point P176 (-17.5984, -33.6793)
  point P177 (-17.3204, -33.8231)
  point P178 (-17.1828, -33.8932)
  point P179 (-16.9031, -34.0336)
  point P180 (-15.4453, -33.5035)
  point P181 (-14.9017, -34.9563)
  point P182 (-14.6133, -35.0778)
  point P183 (-14.4706, -35.1369)
  point P184 (-14.1807, -35.2549)
  point P185 (-12.769, -34.612)
  point P186 (-12.1131, -36.0177)
  point P187 (-11.816, -36.1162)
  point P188 (-11.6692, -36.1639)
  point P189 (-11.3709, -36.2588)
  point P190 (-10.0141, -35.5072)
  point P191 (-9.2499, -36.857)
  point P192 (-8.946, -36.932)
  point P193 (-8.7958, -36.968)
  point P194 (-8.4911, -37.0392)
  point P195 (-7.1973, -36.1834)
  point P196 (-6.3296, -37.4691)
  point P197 (-6.0207, -37.52)
  point P198 (-5.8682, -37.5442)
  point P199 (-5.5588, -37.5912)
  dimension "d6" = 360
  constraints: 640 point on circle, 320 centre point, 160 end point, 1 coincident, 1 horizontal, 1202 other
extrude "Extrusion2" add sketch "Sketch2" along normal blind 12 contours A0 A243 A244 A237 A238 A239 A240 A233 A234 A235 A236 A229 A230 A231 A232 A225 A226 A227 A228 A221 A222 A223 A224 A217 A218 A219 A220 A213 A214 A215 A216 A209 A210 A211 A212 A205 A206 A207 A208 A201 A202 A203 A204 A197 A198 A199 A200 A193 A194 A195 A196 A189 A190 A191 A192 A185 A186 A187 A188 A181 A182 A183 A184 A177 A178 A179 A180 A173 A174 A175 A176 A169 A170 A171 A172 A165 A166 A167 A168 A161 A162 A163 A164 A157 A158 A159 A160 A153 A154 A155 A156 A149 A150 A151 A152 A145 A146 A147 A148 A141 A142 A143 A144 A137 A138 A139 A140 A133 A134 A135 A136 A129 A130 A131 A132 A125 A126 A127 A128 A121 A122 A123 A124 A117 A118 A119 A120 A113 A114 A115 A116 A109 A110 A111 A112 A105 A106 A107 A108 A101 A102 A103 A104 A97 A98 A99 A100 A93 A94 A95 A96 A89 A90 A91 A92 A85 A86 A87 A88 A81 A82 A83 A84 A77 A78 A79 A80 A73 A74 A75 A76 A69 A70 A71 A72 A65 A66 A67 A68 A61 A62 A63 A64 A57 A58 A59 A60 A53 A54 A55 A56 A49 A50 A51 A52 A45 A46 A47 A48 A41 A42 A43 A44 A37 A38 A39 A40 A33 A34 A35 A36 A29 A30 A31 A32 A25 A26 A27 A28 A21 A22 A23 A24 A17 A18 A19 A20 A13 A14 A15 A16 A9 A10 A11 A12 A5 A6 A7 A8 A1 A3 A4 A2 A317 A318 A319 A320 A313 A314 A315 A316 A309 A310 A311 A312 A305 A306 A307 A308 A301 A302 A303 A304 A297 A298 A299 A300 A293 A294 A295 A296 A289 A290 A291 A292 A285 A286 A287 A288 A281 A282 A283 A284 A277 A278 A279 A280 A273 A274 A275 A276 A269 A270 A271 A272 A265 A266 A267 A268 A261 A262 A263 A264 A257 A258 A259 A260 A253 A254 A255 A256 A249 A250 A251 A252 A245 A246 A247 A248 A241 A242
sketch "Sketch3" plane through (0, 14, 0) normal (0, 1, 0) x (1, 0, 0)
  circle A0 centre (0, 0) radius 5
  circle A1 centre (0, 0) radius 22.5
  line L0 (0, 32.3696) -> (0, -28.9406)
  circle A2 centre (0, 22.5) radius 5
  circle A3 centre (22.5, 0) radius 5
  circle A4 centre (0, -22.5) radius 5
  line L1 (-27.5, 0) -> (-29.5, 0)
  line L2 (-29.5, 0) -> (-29.5, 1)
  line L3 (-29.5, 1) -> (-27.399, 1)
  line L4 (-15.5, 1) -> (-15.5, -1)
  line L5 (-29.5, -1) -> (-29.5, 1)
  line L6 (-30.0379, 0) -> (-29.5, 0)
  line L7 (-17.5, 0) -> (29.9007, 0)
  line L8 (-15.5, -1) -> (-17.601, -1)
  line L9 (-27.399, -1) -> (-29.5, -1)
  line L10 (-29.5, 1) -> (-27.399, 1)
  line L11 (-17.601, 1) -> (-15.5, 1)
  arc A5 (-27.399, -1) -> (-17.601, -1) centre (-22.5, 0) ccw
  arc A6 (-17.601, 1) -> (-27.399, 1) centre (-22.5, 0) ccw
  line L12 (-7, 23.5) -> (-4.899, 23.5)
  line L13 (7, 23.5) -> (7, 21.5)
  line L14 (-7, 21.5) -> (-7, 23.5)
  line L15 (7, 21.5) -> (4.899, 21.5)
  line L16 (-4.899, 21.5) -> (-7, 21.5)
  line L17 (4.899, 23.5) -> (7, 23.5)
  line L18 (-7, -21.5) -> (-4.899, -21.5)
  line L19 (7, -21.5) -> (7, -23.5)
  line L20 (-7, -23.5) -> (-7, -21.5)
  line L21 (7, -23.5) -> (4.899, -23.5)
  line L22 (-4.899, -23.5) -> (-7, -23.5)
  line L23 (4.899, -21.5) -> (7, -21.5)
  line L24 (15.5, 1) -> (17.601, 1)
  line L25 (29.5, 1) -> (29.5, -1)
  line L26 (15.5, -1) -> (15.5, 1)
  line L27 (29.5, -1) -> (27.399, -1)
  line L28 (17.601, -1) -> (15.5, -1)
  line L29 (27.399, 1) -> (29.5, 1)
  line L30 (-7, 1) -> (-4.899, 1)
  line L31 (7, 1) -> (7, -1)
  line L32 (-7, -1) -> (-7, 1)
  line L33 (7, -1) -> (4.899, -1)
  line L34 (-4.899, -1) -> (-7, -1)
  line L35 (4.899, 1) -> (7, 1)
  dimension "d10" = 10
  dimension "d11" = 45
  dimension "d13" = 10
  dimension "d14" = 10
  dimension "d15" = 10
  dimension "d41" = 1
  dimension "d43" = 2
  dimension "d44" = 2
  dimension "d45" = 2
  dimension "d46" = 2
  dimension "d47" = 2
  constraints: 72 end point, 18 parallel, 9 horizontal, 8 point on circle, 7 centre point, 7 perpendicular, 3 point on line, 2 coincident, 1 midpoint, 1 vertical
  measures "d10" diameter of A0
  measures "d11" diameter of A1
  measures "d13" diameter of A2
  measures "d14" diameter of A3
  measures "d15" diameter of A4
  measures "d41" distance of L1.end L2.end
  measures "d43" distance of L4.start L4.end
  measures "d44" distance of L13.start L15.start
  measures "d45" distance of L19.start L21.start
  measures "d46" distance of L25.start L27.start
  measures "d47" distance of L31.start L33.start
extrude "Extrusion3" cut sketch "Sketch3" against normal through all contours L7 L0 A0 | L7 L31 L33 A0 | A0 L0 L7 | A0 L35 L31 L7 | L7 A0 L0 | L0 A0 L7 | L7 L32 L30 A0 | A0 L34 L32 L7 | L26 L24 A3 L7 | L7 A3 L28 L26 | A2 A1 L0 | L0 A1 A2 | A4 A1 L0 | L0 A1 A4 | L7 A1 A3 | A3 A1 L7 | L0 A2 A1 | A1 A2 L0 | L16 A1 A2 | A2 A1 L15 | L0 A4 A1 | A1 A4 L0 | L23 A1 A4 | A4 A1 L18 | L4 L8 A5 A1 A6 L11 | L7 A3 A1 | A1 A3 L7 | A2 L17 L13 L15 A1 | A1 L16 L14 L12 A2 | A4 L22 L20 L18 A1 | A1 L23 L19 L21 A4 | L7 L25 L27 A3 | A3 L29 L25 L7 | A1 A5 L9 L5 L2 L3 A6
sketch "Sketch4" plane through (0, 0, 0) normal (0, -1, 0) x (1, 0, 0)
  arc A0 (-4.899, -23.5) -> (4.899, -23.5) centre (0, -22.5) ccw projected
  arc A1 (27.399, 1) -> (17.601, 1) centre (22.5, 0) ccw projected
  line L0 (0, -22.5) -> (22.5, 0)
  arc A2 (4.899, 23.5) -> (-4.899, 23.5) centre (0, 22.5) ccw projected
  line L1 (22.5, 0) -> (0, 22.5)
  arc A3 (-17.601, 1) -> (-27.399, 1) centre (-22.5, 0) ccw projected
  line L2 (0, 22.5) -> (-22.5, 0)
  line L3 (-22.5, 0) -> (0, -22.5)
  line L4 (0, 0) -> (-14.1421, -14.1421)
  line L5 (0, 0) -> (14.1421, -14.1421)
  line L6 (0, 0) -> (14.1421, 14.1421)
  line L7 (0, 0) -> (-14.1421, 14.1421)
  circle A4 centre (11.25, -11.25) radius 1.5
  circle A5 centre (-11.25, -11.25) radius 1.5
  circle A6 centre (-11.25, 11.25) radius 1.5
  circle A7 centre (11.25, 11.25) radius 1.5
  dimension "d18" = 20
  dimension "d21" = 360
  dimension "d23" = 3
  dimension "d26" = 3
  dimension "d29" = 3
  dimension "d32" = 3
  constraints: 16 end point, 4 centre point, 3 perpendicular, 2 coincident, 1 midpoint, 1 point on line, 11 other
  measures "d18" distance of L4.start L4.end
  measures "d23" diameter of A4
  measures "d26" diameter of A5
  measures "d29" diameter of A6
  measures "d32" diameter of A7
hole "Hole1" at (11.25, 0, -11.25) at (-11.25, 0, -11.25) at (-11.25, 0, 11.25) at (11.25, 0, 11.25) direction (0, 1, 0) diameter 3 end through all counterbore diameter 5.6 counterbore depth 3.2
fillet "Fillet1" radius 1 20 edges at (-29.5, 7, -1) (-29.5, 7, 1) (-15.5, 7, -1) (-15.5, 7, 1) (-7, 7, 1) (-7, 7, -1) (7, 7, -1) (7, 7, 1) (-7, 7, 23.5) (-7, 7, 21.5) (7, 7, 21.5) (7, 7, 23.5) (-7, 7, -23.5) (-7, 7, -21.5) (7, 7, -23.5) (7, 7, -21.5) (15.5, 7, -1) (15.5, 7, 1) (29.5, 7, -1) (29.5, 7, 1)
body "Solid1"
